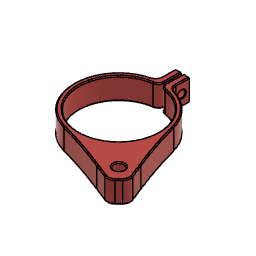
230608 CBR piston dial gauge mounting (Autodesk Fusion 360 design; units mm, degrees)
Autodesk Fusion 360 part; units mm, degrees
sketch "piston ref" plane through (0, 0, 0) normal (0, 1, 0) x (1, 0, 0)
  circle A0 centre (0, 0) radius 25.35
  circle A1 centre (0, 0) radius 25.55 construction
  dimension "d1" = 50.7
  dimension "d2" = 0.2
  dimension "d3" = 51.1
  constraint coincident A0.centre A1.centre
  measures "d1" diameter of A0
  measures "d3" diameter of A1
extrude "Extrude1" add sketch "piston ref" along normal blind 80 makes body 1
sketch "ring mounting" plane through (0, 0, 0) normal (0, 1, 0) x (1, 0, 0)
  circle A0 centre (0, 0) radius 25.55
  line L0 (0, 0) -> (0, 55) construction
  line L1 (0.9964, 28.5326) -> (1.4053, 40.2439)
  line L2 (0, 25.55) -> (0, 40.2684)
  line L3 (0, 40.2684) -> (-4, 40.2684)
  line L4 (-4, 40.2684) -> (-4, 31.5516)
  line L5 (1.4053, 40.2439) -> (5.4029, 40.1043)
  line L6 (5.4029, 40.1043) -> (5.0987, 31.3928)
  line L7 (0.9964, 28.5326) -> (0.8917, 25.5344)
  arc A1 (-7.0169, 27.6743) -> (-4, 31.5516) centre (-8, 31.5516) ccw
  arc A2 (5.0987, 31.3928) -> (7.9784, 27.4125) centre (9.0963, 31.2532) ccw
  line L8 (0, 0) -> (60.8712, -60.8712) construction
  line L9 (0, 0) -> (0, -44) construction
  line L10 (0, -28.55) -> (35.7442, -42.8153)
  line L11 (35.7442, -42.8153) -> (42.8153, -35.7442)
  line L12 (42.8153, -35.7442) -> (28.55, 0)
  line L13 (0, 0) -> (44, 0) construction
  arc A3 (-7.0169, 27.6743) -> (0, -28.55) centre (0, 0) ccw
  arc A4 (28.55, 0) -> (7.9784, 27.4125) centre (0, 0) ccw
  line L14 (18.0666, -18.0666) -> (1.7407, -34.3924) construction
  circle A5 centre (32.2087, -32.2087) radius 3.3
  line L15 (32.2087, -32.2087) -> (47.6032, -16.8142) construction
  point P0 (-4, 28.2684)
  point P1 (4.9841, 28.1116)
  dimension "d8" = 2
  dimension "d9" = 3
  dimension "d10" = 4
  dimension "d11" = 4
  dimension "d14" = 12
  dimension "d15" = 12
  dimension "d16" = 4
  dimension "d31" = 135
  dimension "d32" = 30
  dimension "d33" = 6.6
  dimension "d34" = 10
  dimension "d55" = 20
  constraint coincident A0.centre L0.start
  constraint vertical L0
  constraint coincident L1.start A3
  constraint coincident A0.centre L1
  constraint coincident L0 L2.start
  constraint parallel L0 L2
  constraint perpendicular L2 L3
  constraint perpendicular L3 L4
  constraint concentric A0 A3
  constraint perpendicular L1 L5
  constraint perpendicular L5 L6
  constraint coincident A0 L7.end
  constraint parallel L1 L7
  constraint coincident A0 L2.start
  constraint coincident P0 L4
  constraint coincident P0 A3
  constraint tangent L4 A1
  constraint tangent A1 A3
  constraint coincident P1 L6
  constraint coincident P1 A3
  constraint tangent L6 A2
  constraint tangent A2 A3
  constraint equal A1 A2
  constraint vertical L9
  constraint coincident L9 L10.start
  constraint perpendicular L8 L11
  constraint perpendicular L9 L13
  constraint coincident L12.end L13
  constraint coincident L12.end A3
  constraint concentric A3 A4
  constraint symmetric L8 L10 L12
  constraint coincident A0 L14.start
  constraint coincident L8 L14.start
  constraint tangent A0 L14
  constraint coincident L8 A5.centre
  constraint coincident A5.centre L15.start
  measures "d8" angle of L0 L1
  measures "d9" distance of A0 A3
  measures "d10" distance of L2.end L3.end
  measures "d11" distance of L1.end L5.end
  measures "d14" distance of L3 P0
  measures "d15" distance of L5 P1
  measures "d16" radius of A1
  measures "d31" angle of L0 L8
  measures "d32" distance of L11 L14
  measures "d33" diameter of A5
  measures "d34" distance of L10.end L11.end
  measures "d55" distance of L14 L15
extrude "Extrude2" add sketch "ring mounting" along normal blind 14 separate body contours A0 L1 L2 L3 L4 L5 L6 L7 A1 A2 L10 L11 L12 A3 A4 makes body 2
sketch "heat insert hole" plane through (3.9976, 0, 0.1396) normal (0.999391, 0, 0.034899) x (0.034899, 0, -0.999391)
  line L0 (31.5516, 0) -> (40.2684, 0)
  line L1 (40.2684, 0) -> (40.2684, 14)
  line L2 (40.2684, 14) -> (31.5516, 14)
  line L3 (31.5516, 14) -> (31.5516, 0)
  circle A0 centre (35.2684, 7) radius 2.3
  line L4 (40.2684, 7) -> (31.5516, 7) construction
  line L5 (35.2684, 14) -> (35.2684, 0) construction
  dimension "d19" = 4.6
  dimension "d30" = 5
  constraint midpoint L1 L4.start
  constraint midpoint L3 L4.end
  constraint midpoint A0.centre L5
  constraint coincident L2 L5.start
  constraint coincident L0 L5.end
  measures "d19" diameter of A0
  measures "d30" distance of L1 L5
extrude "Extrude3" cut sketch "heat insert hole" against normal blind 4 contours A0 bodies 2
chamfer "Chamfer1" distance 0.4 angle 45 1 edges at (5.1536, 7.8317, -32.9643) on bodies 2
sketch "M3 hole" plane through (-4, 0, 0) normal (-1, 0, 0) x (0, 0, 1)
  line L0 (-40.2684, 0) -> (-31.5516, 0)
  line L1 (-31.5516, 0) -> (-31.5516, 14)
  line L2 (-31.5516, 14) -> (-40.2684, 14)
  line L3 (-40.2684, 14) -> (-40.2684, 0)
  ellipse E0 centre (-35.1073, 7) end of major axis (-35.1073, 9.3) minor radius 2.2986
  circle A0 centre (-35.1073, 7) radius 1.65
  dimension "d24" = 3.3
  constraint concentric E0 A0
  measures "d24" diameter of A0
extrude "Extrude4" cut sketch "M3 hole" against normal blind 4 contours A0 bodies 2
fillet "Fillet1" radius 4 2 edges at (0, 7, -25.55) (0.8917, 7, -25.5344) on bodies 2
chamfer "Chamfer2" distance 0.4 angle 45 4 edges at (5.4029, 7, -40.1043) (1.4053, 7, -40.2439) (0, 7, -40.2684) (-4, 7, -40.2684) on bodies 2
fillet "Fillet2" radius 5 2 edges at (35.7442, 7, 42.8153) (42.8153, 7, 35.7442) on bodies 2
fillet "Fillet3" radius 300 2 edges at (28.55, 7, 0) (0, 7, 28.55) on bodies 2
chamfer "Chamfer6" distance 0.6 angle 45 2 faces at (28.301, 14, 19.6974) (28.301, 0, 19.6974) on bodies 2
chamfer "Chamfer5" [suppressed]
hidden bodies 1
equation "ringDistance = 20 mm"
named bodies: "piston", "ring mounting w ear"
